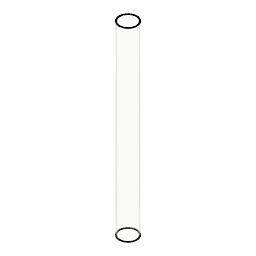
Tubo (Autodesk Fusion 360 design; units mm, degrees)
part number: 2025-09-05-15-36-02-729
Autodesk Fusion 360 part; units mm, degrees
sketch "Boceto1" plane through (0, 0, 0) normal (0, 0, 1) x (1, 0, 0)
  circle A0 centre (0, 0) radius 40.2
  dimension "d1" = 80.4
  constraint coincident A0.centre origin
  measures "d1" diameter of A0
extrude "Extruir1" add sketch "Boceto1" along normal blind 840
sketch "Boceto2" plane through (0, 0, 840) normal (0, 0, 1) x (-1, 0, 0)
  circle A0 centre (0, 0) radius 40.2
  circle A1 centre (0, 0) radius 37.3
  dimension "d4" = 74.6
  constraint coincident A0.centre A1.centre
  measures "d4" diameter of A1
extrude "Extruir2" cut sketch "Boceto2" against normal blind 880 contours A1
